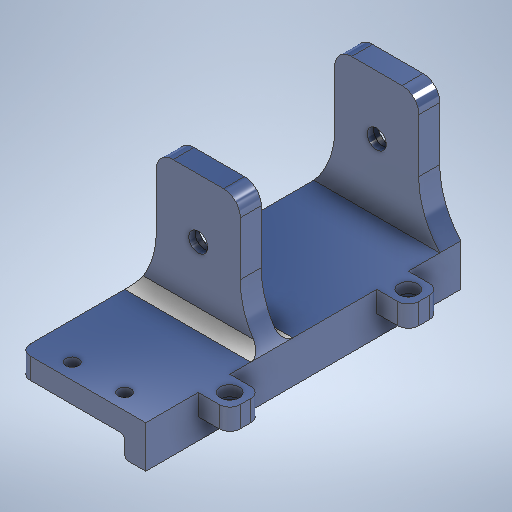
# Autodesk Inventor part: soporte_inferior
Saved by Autodesk Inventor 2026 (Build 300175050, 175E)
## iProperties
Created: 2025-06-30
Part Number: soporte_inferior
Material: Genérico
Document SubType Name: Modeling
Designer: piero
Density: 1 g/cm^3
Appearance: Valor por defecto
Author: piero
Autodesk Inventor part; units mm, degrees
ref_plane "YZ Plane" through (0, 0, 0) normal (1, 0, 0) x (0, 1, 0)
ref_plane "XZ Plane" through (0, 0, 0) normal (0, 1, 0) x (-1, 0, 0)
ref_plane "XY Plane" through (0, 0, 0) normal (0, 0, 1) x (1, 0, 0)
sketch "Boceto1" plane through (0, 0, 0) normal (0, 1, 0) x (-1, 0, 0)
  line L0 (0, 0) -> (80, 0)
  line L1 (80, 0) -> (80, -150)
  line L2 (80, -150) -> (0, -150)
  line L3 (0, -150) -> (0, 0)
  line L4 (80, -150) -> (0, -150)
  line L5 (0, -150) -> (0, -140)
  line L6 (0, -140) -> (80, -140)
  line L7 (80, -140) -> (80, -150)
  line L8 (80, -65) -> (0, -65)
  line L9 (0, -65) -> (0, -55)
  line L10 (0, -55) -> (80, -55)
  line L11 (80, -55) -> (80, -65)
  line L12 (80, -25) -> (0, -25)
  line L13 (0, -25) -> (0, -15)
  line L14 (0, -15) -> (80, -15)
  line L15 (80, -15) -> (80, -25)
  point P0 (0, -65)
  point P1 (0, -15)
  point P2 (0, -25)
  point P3 (0, -55)
  point P4 (80, -55)
  dimension "d0" = 80
  dimension "d1" = 150
  dimension "d4" = 80
  dimension "d5" = 10
  dimension "d6" = 80
  dimension "d7" = 10
  dimension "d8" = 80
  dimension "d9" = 10
  dimension "d17" = 75
  dimension "d19" = 30
  constraints: 32 end point, 8 parallel, 4 horizontal, 4 perpendicular, 2 point on line
  measures "d0" distance of L1.end L2.end
  measures "d1" distance of L0.end L1.end
  measures "d4" distance of L5.end L6.end
  measures "d5" distance of L4.end L5.end
  measures "d6" distance of L9.end L10.end
  measures "d7" distance of L8.end L9.end
  measures "d8" distance of L13.end L14.end
  measures "d9" distance of L12.end L13.end
  measures "d17" distance between parallel lines of L8 L6
  measures "d19" distance between parallel lines of L10 L12
extrude "Extrusión1" add sketch "Boceto1" along normal blind 10 contours L0 L1 L14 L3 | L12 L1 L10 L3 | L8 L1 L6 L3
extrude "Extrusión2" add sketch "Boceto1" along normal blind 70 contours L14 L1 L12 L3 | L10 L1 L8 L3 | L6 L1 L2 L3
sketch "Boceto3" plane through (0, 0, -150) normal (0, 0, -1) x (-1, 0, 0)
  circle A0 centre (40, 42) radius 4.5
  line L0 (0, 0) -> (0, 70) projected
  line L1 (0, 70) -> (80, 70) projected
  line L2 (80, 10) -> (0, 10) projected
  circle A1 centre (40, 42) radius 11
  dimension "d12" = 9
  dimension "d13" = 40
  dimension "d18" = 32
  dimension "d54" = 22
  constraints: 2 centre point, 1 coincident
  measures "d12" diameter of A0
  measures "d13" distance from line of A0.centre L0
  measures "d18" distance from line of L2 A0.centre
  measures "d54" diameter of A1
extrude "Extrusión3" cut sketch "Boceto3" against normal blind 10 contours A0
sketch "Boceto4" plane through (-80, 10, -15) normal (0, 0, 1) x (1, 0, 0)
  circle A0 centre (40, 32) radius 4.5 projected
  circle A1 centre (40, 32) radius 4
  circle A2 centre (40, 32) radius 12.5
  circle A3 centre (24.5, 47.4996) radius 1.5
  circle A4 centre (55.5, 47.4996) radius 1.5
  circle A5 centre (24.5009, 16.4996) radius 1.5
  circle A6 centre (55.4991, 16.4996) radius 1.5
  point P0 (80, -10)
  dimension "d20" = 8
  dimension "d21" = 25
  dimension "d26" = 3
  dimension "d27" = 21.92
  dimension "d28" = 3
  dimension "d29" = 21.92
  dimension "d30" = 3
  dimension "d31" = 3
  dimension "d32" = 21.92
  dimension "d33" = 21.92
  dimension "d47" = 0
  dimension "d48" = 31
  dimension "d51" = 0
  dimension "d53" = 31
  constraints: 6 centre point, 2 coincident
  measures "d20" diameter of A1
  measures "d21" diameter of A2
  measures "d26" diameter of A3
  measures "d27" distance of A2.centre A3.centre
  measures "d28" diameter of A4
  measures "d29" distance of A2.centre A4.centre
  measures "d30" diameter of A5
  measures "d31" diameter of A6
  measures "d32" distance of A2.centre A5.centre
  measures "d33" distance of A1.centre A6.centre
  measures "d47" vertical distance of A4.centre A3.centre
  measures "d48" distance of A4.centre A3.centre
  measures "d51" vertical distance of A6.centre A5.centre
  measures "d53" distance of A5.centre A3.centre
extrude "Extrusión4" cut sketch "Boceto4" against normal blind 10 contours A1
extrude "Extrusión6" cut sketch "Boceto4" against normal blind 8 contours A0 | A2
sketch "Boceto5" plane through (0, 10, -65) normal (0, 0, -1) x (-1, 0, 0)
  circle A0 centre (40, 32) radius 4 projected
  circle A1 centre (40, 32) radius 4.5
  point P0 (0, -10)
  dimension "d44" = 9
  constraints: 1 centre point, 1 coincident
  measures "d44" diameter of A1
extrude "Extrusión7" cut sketch "Boceto5" against normal blind 10 contours A0 | A1
sketch "Boceto7" plane through (-80, 10, -15) normal (0, 0, 1) x (1, 0, 0)
  line L0 (0, -10) -> (0, 60) projected
  line L1 (0, 0) -> (80, 0) projected
  line L2 (0, 60) -> (20, 60)
  line L3 (20, 60) -> (20, 0)
  line L4 (20, 0) -> (0, 0)
  line L5 (0, 0) -> (0, 60)
  line L6 (80, 60) -> (60, 60)
  line L7 (60, 60) -> (60, 0)
  line L8 (60, 0) -> (80, 0)
  line L9 (80, 0) -> (80, 60)
  point P0 (80, -10)
  dimension "d58" = 20
  dimension "d59" = 20
  constraints: 16 end point, 4 parallel, 3 point on line, 2 horizontal, 2 perpendicular
  measures "d58" distance of L3.end L4.end
  measures "d59" distance of L8.end L7.end
extrude "Extrusión9" cut sketch "Boceto7" against normal blind 150
fillet "Empalme3" radius 8 1 edges at (-60, 70, -60)
fillet "Empalme4" radius 8 1 edges at (-20, 70, -60)
fillet "Empalme5" radius 8 1 edges at (-60, 70, -145)
fillet "Empalme6" radius 8 1 edges at (-20, 70, -145)
sketch "Boceto8" plane through (-20, 10, -65) normal (0, 0, -1) x (-1, 0, 0)
  circle A0 centre (20, 32) radius 11 projected
  circle A1 centre (20, 32) radius 11
  point P0 (-20, -10)
  dimension "d68" = 22
  constraints: 1 centre point, 1 coincident
  measures "d68" diameter of A1
extrude "Extrusión10" cut sketch "Boceto8" against normal blind 7
sketch "Boceto9" plane through (-80, 0, 0) normal (0, 0, 1) x (1, 0, 0)
  line L0 (0, 0) -> (80, 0) projected
  line L1 (0, 10) -> (10, 10)
  line L2 (10, 10) -> (10, 0)
  line L3 (10, 0) -> (0, 0)
  line L4 (0, 0) -> (0, 10)
  line L5 (0, 10) -> (80, 10) projected
  line L6 (80, 10) -> (70, 10)
  line L7 (70, 10) -> (70, 0)
  line L8 (70, 0) -> (80, 0)
  line L9 (80, 0) -> (80, 10)
  dimension "d71" = 10
  dimension "d72" = 10
  constraints: 16 end point, 4 parallel, 2 horizontal, 2 perpendicular, 2 point on line
  measures "d71" distance of L2.end L3.end
  measures "d72" distance of L8.end L7.end
extrude "Extrusión11" cut sketch "Boceto9" against normal blind 150 contours L4 L1 L2 L0 | L7 L5 L9 L0
sketch "Boceto10" plane through (-60, 10, -15) normal (0, 0, 1) x (1, 0, 0)
  line L0 (0, 52) -> (0, 0) projected
  line L1 (0, 0) -> (40, 0)
  line L2 (40, 0) -> (40, 60)
  line L3 (40, 60) -> (0, 60)
  line L4 (0, 60) -> (0, 0)
  point P0 (60, -10)
  dimension "d75" = 40
  dimension "d76" = 60
  constraints: 8 end point, 2 parallel, 1 horizontal, 1 perpendicular
  measures "d75" distance of L3.end L2.end
  measures "d76" distance of L2.end L1.end
extrude "Extrusión12" cut sketch "Boceto10" against normal blind 10
sketch "Boceto12" plane through (0, 10, 0) normal (0, 1, 0) x (1, 0, 0)
  line L0 (-10, 0) -> (-10, 150) projected
  line L1 (-10, 125) -> (5, 125)
  line L2 (5, 125) -> (5, 110)
  line L3 (5, 110) -> (-10, 110)
  line L4 (-10, 110) -> (-10, 125)
  line L5 (-10, 40) -> (5, 40)
  line L6 (5, 40) -> (5, 25)
  line L7 (5, 25) -> (-10, 25)
  line L8 (-10, 25) -> (-10, 40)
  line L9 (-20, 150) -> (-10, 150) projected
  circle A0 centre (-2.5, 117.5) radius 3
  circle A1 centre (-2.5, 32.5) radius 3
  circle A2 centre (-2.5, 32.5) radius 4.5
  circle A3 centre (-2.5, 117.5) radius 4.5
  point P0 (0, 0)
  point P1 (-2.5, 125)
  point P2 (-15, 150)
  point P3 (-2.5, 25)
  dimension "d85" = 15
  dimension "d86" = 15
  dimension "d87" = 15
  dimension "d88" = 15
  dimension "d89" = 25
  dimension "d90" = 25
  dimension "d109" = 6
  dimension "d110" = 6
  dimension "d133" = 9
  dimension "d134" = 9
  constraints: 16 end point, 4 centre point, 4 parallel, 3 midpoint, 2 coincident, 2 horizontal, 2 perpendicular, 2 point on line
  measures "d85" distance of L2.end L3.end
  measures "d86" distance of L1.end L2.end
  measures "d87" distance of L6.end L7.end
  measures "d88" distance of L5.end L6.end
  measures "d89" vertical distance of point (-2.5, 125) point (-15, 150)
  measures "d90" vertical distance of point (-2.5, 25) L0.start
  measures "d109" diameter of A0
  measures "d110" diameter of A1
  measures "d133" diameter of A2
  measures "d134" diameter of A3
extrude "Extrusión14" add sketch "Boceto12" against normal blind 10 contours L0 L5 L6 L7 | L0 L1 L2 L3 | A2 | A3
sketch "Boceto13" plane through (0, 0, 0) normal (0, -1, 0) x (1, 0, 0)
  line L0 (-70, 0) -> (-10, 0) projected
  line L1 (-10, -150) -> (-70, -150) projected
  line L2 (-10, 0) -> (-20, 0)
  line L3 (-20, 0) -> (-20, -150)
  line L4 (-20, -150) -> (-10, -150)
  line L5 (-10, -150) -> (-10, 0)
  point P0 (0, 0)
  dimension "d98" = 10
  constraints: 8 end point, 2 parallel, 1 horizontal, 1 perpendicular, 1 point on line
  measures "d98" distance of L4.end L3.end
extrude "Extrusión15" add sketch "Boceto13" along normal blind 10
fillet "Empalme7" radius 5 4 edges at (5, 5, -25) (5, 5, -40) (5, 5, -110) (5, 5, -125)
fillet "Empalme8" radius 2 2 edges at (-20, -10, -75) (-20, 0, -75)
sketch "Boceto15" plane through (0, 10, 0) normal (0, 1, 0) x (1, 0, 0)
  line L0 (-10, 25) -> (0, 25) projected
  line L1 (-10, 25) -> (-70, 25)
  line L2 (-70, 150) -> (-70, 0) projected
  line L3 (-10, 0) -> (-10, 25) projected
  line L4 (-60, 55) -> (-60, 65) projected
  line L5 (-20, 0) -> (-20, 150) projected
  line L6 (-20, 40) -> (-20, 8.1817)
  circle A0 centre (-27.5, 7.5) radius 3
  circle A1 centre (-52.5, 7.5) radius 3
  line L7 (-70, 0) -> (-10, 0) projected
  point P0 (0, 0)
  point P1 (-70, 145)
  point P2 (-70, 5)
  point P3 (-65, 0)
  dimension "d127" = 6
  dimension "d128" = 7.5
  dimension "d130" = 6
  dimension "d137" = 7.5
  dimension "d138" = 7.5
  constraints: 4 end point, 3 point on line, 2 centre point, 1 horizontal
  measures "d127" diameter of A0
  measures "d128" distance from line of L5 A0.centre
  measures "d130" diameter of A1
  measures "d137" distance from line of A1.centre L7
  measures "d138" distance from line of L7 A0.centre
extrude "Extrusión17" cut sketch "Boceto15" against normal blind 10 contours A0 | A1
extrude "Extrusión18" cut sketch "Boceto12" against normal blind 5 contours A2 | A3
fillet "Empalme10" radius 40 4 edges at (-20, 10, -60) (-20, 10, -145) (-60, 10, -60) (-60, 10, -145)
fillet "Empalme11" radius 5 1 edges at (-70, 5, 0)
sketch "Boceto16" plane through (-28, 70, -150) normal (0, 0, -1) x (-1, 0, 0)
  circle A0 centre (12, -28) radius 4.5 projected
  circle A1 centre (12, -28) radius 4
  circle A2 centre (12, -28) radius 11
  point P0 (-28, -70)
  dimension "d141" = 8
  dimension "d142" = 22
  constraints: 2 centre point, 2 coincident
  measures "d141" diameter of A1
  measures "d142" diameter of A2
extrude "Extrusión19" cut sketch "Boceto16" against normal blind 7 contours A0 | A2
fillet "Empalme12" radius 5 1 edges at (-40, 10, -55)
fillet "Empalme13" radius 5 1 edges at (-40, 10, -65)
